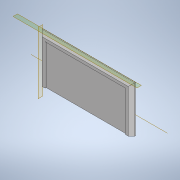
# Autodesk Inventor part: Top Base
Saved by Autodesk Inventor 2022 (Build 260153000, 153)
## iProperties
Created: 2022-04-03
Part Number: Top Base
Material: Generic
Document SubType Name: Modeling
Designer: Nick
Density: 1 g/cm^3
Appearance: Default
Author: Nick
Autodesk Inventor part; units mm, degrees
ref_plane "YZ Plane" through (0, 0, 0) normal (1, 0, 0) x (0, 1, 0)
ref_plane "XZ Plane" through (0, 0, 0) normal (0, 1, 0) x (-1, 0, 0)
ref_plane "XY Plane" through (0, 0, 0) normal (0, 0, 1) x (1, 0, 0)
sketch "Sketch1" plane through (-152.4, -88.9, 0) normal (0, 0, 1) x (1, 0, 0)
  line L0 (2.3554, 30.5524) -> (256.3554, 30.5524)
  line L1 (256.3554, 30.5524) -> (256.3554, 157.5524)
  line L2 (256.3554, 157.5524) -> (2.3554, 157.5524)
  line L3 (2.3554, 157.5524) -> (2.3554, 30.5524)
  line L4 (-16.6946, 30.5524) -> (275.4054, 30.5524)
  line L5 (275.4054, 30.5524) -> (275.4054, 176.6024)
  line L6 (275.4054, 176.6024) -> (-16.6946, 176.6024)
  line L7 (-16.6946, 176.6024) -> (-16.6946, 30.5524)
  point P0 (129.3554, 30.5524)
  point P1 (256.3554, 30.5524)
  point P2 (2.3554, 30.5524)
  dimension "d2" = 254
  dimension "d3" = 127
  dimension "d0" = 19.05
  dimension "d1" = 19.05
  constraints: 16 end point, 4 parallel, 2 horizontal, 2 midpoint, 2 perpendicular
  measures "d2" distance of L2.end L1.end
  measures "d3" distance of L1.end L0.end
  measures "d0" distance between parallel lines of L7 L3
  measures "d1" distance between parallel lines of L6 L2
extrude "Extrusion1" add sketch "Sketch1" along normal blind 12.7 contours L4 L7 L6 L5 L1 L2 L3
extrude "Extrusion2" add sketch "Sketch1" along normal blind 9.525 contours L3 L2 L1 L0
chamfer "Chamfer1" distance 10.16 angle 45 3 edges at (-169.0946, 14.6774, 12.7) (-23.0446, 87.7024, 12.7) (123.0054, 14.6774, 12.7)
ref_plane "Work Plane1" through (-169.0946, 87.7024, 0) normal (1, 0, 0) x (0, -1, 0)
sketch "Sketch2" plane through (-169.0946, 87.7024, 0) normal (1, 0, 0) x (0, -1, 0)
  line L0 (0, 0) -> (146.05, 0) projected
  point P0 (88.9, 0)
  point P1 (88.9, 0)
  dimension "d17" = 88.9
  constraints: 1 coincident, 1 point on line
  measures "d17" distance of point (88.9, 0) L0.start
ref_plane "Work Plane2" through (123.0054, 87.7024, 0) normal (0, -1, 0) x (-1, 0, 0)
equation "\"d1\" = d0"
body "Solid1"
